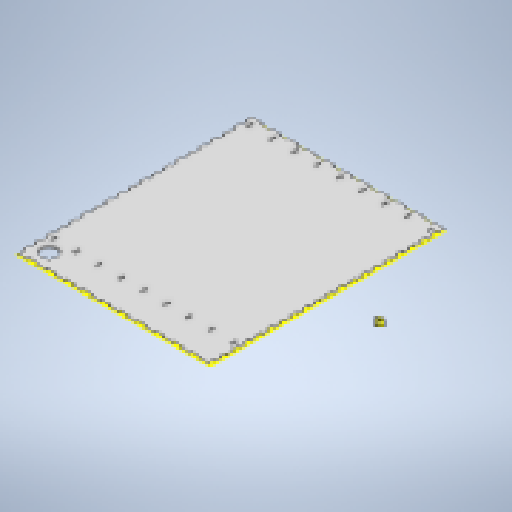
# Autodesk Inventor part: LedBoard
Saved by Autodesk Inventor 2024 (Build 280153000, 153)
## iProperties
Created: 2023-07-20
Part Number: LedBoard
Material: Generic
Document SubType Name: Modeling
Designer: Bruno
Density: 1 g/cm^3
Appearance: Default
Author: Bruno
Autodesk Inventor part; units mm, degrees
ref_plane "YZ Plane" through (0, 0, 0) normal (1, 0, 0) x (0, 1, 0)
ref_plane "XZ Plane" through (0, 0, 0) normal (0, 1, 0) x (-1, 0, 0)
ref_plane "XY Plane" through (0, 0, 0) normal (0, 0, 1) x (1, 0, 0)
sketch "Sketch1" plane through (0, 0, 0) normal (0, 1, 0) x (-1, 0, 0)
  line L0 (378.2704, -187.5) -> (378.2704, 177.5) projected
  line L1 (78.2704, -187.5) -> (378.2704, -187.5) projected
  line L2 (78.2704, 177.5) -> (78.2704, -187.5) projected
  line L3 (378.2704, 177.5) -> (78.2704, 177.5) projected
  line L4 (378.2704, 168.375) -> (378.2704, 177.5) projected
  line L5 (378.2704, 177.5) -> (375.2704, 177.5) projected
  line L6 (375.2704, 168.375) -> (375.2704, 177.5) projected
  line L7 (378.2704, 168.375) -> (375.2704, 168.375) projected
  line L8 (378.2704, 150.125) -> (378.2704, 159.25) projected
  line L9 (378.2704, 159.25) -> (375.2704, 159.25) projected
  line L10 (375.2704, 150.125) -> (375.2704, 159.25) projected
  line L11 (378.2704, 150.125) -> (375.2704, 150.125) projected
  line L12 (378.2704, 131.875) -> (378.2704, 141) projected
  line L13 (378.2704, 141) -> (375.2704, 141) projected
  line L14 (375.2704, 131.875) -> (375.2704, 141) projected
  line L15 (378.2704, 131.875) -> (375.2704, 131.875) projected
  line L16 (378.2704, 113.625) -> (378.2704, 122.75) projected
  line L17 (378.2704, 122.75) -> (375.2704, 122.75) projected
  line L18 (375.2704, 113.625) -> (375.2704, 122.75) projected
  line L19 (378.2704, 113.625) -> (375.2704, 113.625) projected
  line L20 (378.2704, 95.375) -> (378.2704, 104.5) projected
  line L21 (378.2704, 104.5) -> (375.2704, 104.5) projected
  line L22 (375.2704, 95.375) -> (375.2704, 104.5) projected
  line L23 (378.2704, 95.375) -> (375.2704, 95.375) projected
  line L24 (378.2704, 77.125) -> (378.2704, 86.25) projected
  line L25 (378.2704, 86.25) -> (375.2704, 86.25) projected
  line L26 (375.2704, 77.125) -> (375.2704, 86.25) projected
  line L27 (378.2704, 77.125) -> (375.2704, 77.125) projected
  line L28 (378.2704, 58.875) -> (378.2704, 68) projected
  line L29 (378.2704, 68) -> (375.2704, 68) projected
  line L30 (375.2704, 58.875) -> (375.2704, 68) projected
  line L31 (378.2704, 58.875) -> (375.2704, 58.875) projected
  line L32 (378.2704, 4.125) -> (378.2704, 13.25) projected
  line L33 (378.2704, 13.25) -> (375.2704, 13.25) projected
  line L34 (375.2704, 4.125) -> (375.2704, 13.25) projected
  line L35 (378.2704, 4.125) -> (375.2704, 4.125) projected
  line L36 (378.2704, 22.375) -> (378.2704, 31.5) projected
  line L37 (378.2704, 31.5) -> (375.2704, 31.5) projected
  line L38 (375.2704, 22.375) -> (375.2704, 31.5) projected
  line L39 (378.2704, 22.375) -> (375.2704, 22.375) projected
  line L40 (378.2704, 40.625) -> (378.2704, 49.75) projected
  line L41 (378.2704, 49.75) -> (375.2704, 49.75) projected
  line L42 (375.2704, 40.625) -> (375.2704, 49.75) projected
  line L43 (378.2704, 40.625) -> (375.2704, 40.625) projected
  line L44 (378.2704, -87.125) -> (378.2704, -78) projected
  line L45 (378.2704, -78) -> (375.2704, -78) projected
  line L46 (375.2704, -87.125) -> (375.2704, -78) projected
  line L47 (378.2704, -87.125) -> (375.2704, -87.125) projected
  line L48 (378.2704, -68.875) -> (378.2704, -59.75) projected
  line L49 (378.2704, -59.75) -> (375.2704, -59.75) projected
  line L50 (375.2704, -68.875) -> (375.2704, -59.75) projected
  line L51 (378.2704, -68.875) -> (375.2704, -68.875) projected
  line L52 (378.2704, -50.625) -> (378.2704, -41.5) projected
  line L53 (378.2704, -41.5) -> (375.2704, -41.5) projected
  line L54 (375.2704, -50.625) -> (375.2704, -41.5) projected
  line L55 (378.2704, -50.625) -> (375.2704, -50.625) projected
  line L56 (378.2704, -32.375) -> (378.2704, -23.25) projected
  line L57 (378.2704, -23.25) -> (375.2704, -23.25) projected
  line L58 (375.2704, -32.375) -> (375.2704, -23.25) projected
  line L59 (378.2704, -32.375) -> (375.2704, -32.375) projected
  line L60 (378.2704, -14.125) -> (378.2704, -5) projected
  line L61 (378.2704, -5) -> (375.2704, -5) projected
  line L62 (375.2704, -14.125) -> (375.2704, -5) projected
  line L63 (378.2704, -14.125) -> (375.2704, -14.125) projected
  line L64 (378.2704, -178.375) -> (378.2704, -169.25) projected
  line L65 (378.2704, -169.25) -> (375.2704, -169.25) projected
  line L66 (375.2704, -178.375) -> (375.2704, -169.25) projected
  line L67 (378.2704, -178.375) -> (375.2704, -178.375) projected
  line L68 (378.2704, -160.125) -> (378.2704, -151) projected
  line L69 (378.2704, -151) -> (375.2704, -151) projected
  line L70 (375.2704, -160.125) -> (375.2704, -151) projected
  line L71 (378.2704, -160.125) -> (375.2704, -160.125) projected
  line L72 (378.2704, -141.875) -> (378.2704, -132.75) projected
  line L73 (378.2704, -132.75) -> (375.2704, -132.75) projected
  line L74 (375.2704, -141.875) -> (375.2704, -132.75) projected
  line L75 (378.2704, -141.875) -> (375.2704, -141.875) projected
  line L76 (378.2704, -123.625) -> (378.2704, -114.5) projected
  line L77 (378.2704, -114.5) -> (375.2704, -114.5) projected
  line L78 (375.2704, -123.625) -> (375.2704, -114.5) projected
  line L79 (378.2704, -123.625) -> (375.2704, -123.625) projected
  line L80 (378.2704, -105.375) -> (378.2704, -96.25) projected
  line L81 (378.2704, -96.25) -> (375.2704, -96.25) projected
  line L82 (375.2704, -105.375) -> (375.2704, -96.25) projected
  line L83 (378.2704, -105.375) -> (375.2704, -105.375) projected
  line L84 (361.2704, -184.5) -> (347.2704, -184.5) projected
  line L85 (347.2704, -184.5) -> (347.2704, -187.5) projected
  line L86 (361.2704, -187.5) -> (347.2704, -187.5) projected
  line L87 (361.2704, -184.5) -> (361.2704, -187.5) projected
  line L88 (333.2704, -184.5) -> (319.2704, -184.5) projected
  line L89 (319.2704, -184.5) -> (319.2704, -187.5) projected
  line L90 (333.2704, -187.5) -> (319.2704, -187.5) projected
  line L91 (333.2704, -184.5) -> (333.2704, -187.5) projected
  line L92 (305.2704, -184.5) -> (291.2704, -184.5) projected
  line L93 (291.2704, -184.5) -> (291.2704, -187.5) projected
  line L94 (305.2704, -187.5) -> (291.2704, -187.5) projected
  line L95 (305.2704, -184.5) -> (305.2704, -187.5) projected
  line L96 (277.2704, -184.5) -> (263.2704, -184.5) projected
  line L97 (263.2704, -184.5) -> (263.2704, -187.5) projected
  line L98 (277.2704, -187.5) -> (263.2704, -187.5) projected
  line L99 (277.2704, -184.5) -> (277.2704, -187.5) projected
  line L100 (249.2704, -184.5) -> (235.2704, -184.5) projected
  line L101 (235.2704, -184.5) -> (235.2704, -187.5) projected
  line L102 (249.2704, -187.5) -> (235.2704, -187.5) projected
  line L103 (249.2704, -184.5) -> (249.2704, -187.5) projected
  line L104 (221.2704, -184.5) -> (207.2704, -184.5) projected
  line L105 (207.2704, -184.5) -> (207.2704, -187.5) projected
  line L106 (221.2704, -187.5) -> (207.2704, -187.5) projected
  line L107 (221.2704, -184.5) -> (221.2704, -187.5) projected
  line L108 (193.2704, -184.5) -> (179.2704, -184.5) projected
  line L109 (179.2704, -184.5) -> (179.2704, -187.5) projected
  line L110 (193.2704, -187.5) -> (179.2704, -187.5) projected
  line L111 (193.2704, -184.5) -> (193.2704, -187.5) projected
  line L112 (165.2704, -184.5) -> (151.2704, -184.5) projected
  line L113 (151.2704, -184.5) -> (151.2704, -187.5) projected
  line L114 (165.2704, -187.5) -> (151.2704, -187.5) projected
  line L115 (165.2704, -184.5) -> (165.2704, -187.5) projected
  line L116 (137.2704, -184.5) -> (123.2704, -184.5) projected
  line L117 (123.2704, -184.5) -> (123.2704, -187.5) projected
  line L118 (137.2704, -187.5) -> (123.2704, -187.5) projected
  line L119 (137.2704, -184.5) -> (137.2704, -187.5) projected
  line L120 (109.2704, -184.5) -> (95.2704, -184.5) projected
  line L121 (95.2704, -184.5) -> (95.2704, -187.5) projected
  line L122 (109.2704, -187.5) -> (95.2704, -187.5) projected
  line L123 (109.2704, -184.5) -> (109.2704, -187.5) projected
  line L124 (81.2704, -178.375) -> (81.2704, -169.25) projected
  line L125 (81.2704, -169.25) -> (78.2704, -169.25) projected
  line L126 (78.2704, -178.375) -> (78.2704, -169.25) projected
  line L127 (81.2704, -178.375) -> (78.2704, -178.375) projected
  line L128 (81.2704, -160.125) -> (81.2704, -151) projected
  line L129 (81.2704, -151) -> (78.2704, -151) projected
  line L130 (78.2704, -160.125) -> (78.2704, -151) projected
  line L131 (81.2704, -160.125) -> (78.2704, -160.125) projected
  line L132 (81.2704, -141.875) -> (81.2704, -132.75) projected
  line L133 (81.2704, -132.75) -> (78.2704, -132.75) projected
  line L134 (78.2704, -141.875) -> (78.2704, -132.75) projected
  line L135 (81.2704, -141.875) -> (78.2704, -141.875) projected
  line L136 (81.2704, -123.625) -> (81.2704, -114.5) projected
  line L137 (81.2704, -114.5) -> (78.2704, -114.5) projected
  line L138 (78.2704, -123.625) -> (78.2704, -114.5) projected
  line L139 (81.2704, -123.625) -> (78.2704, -123.625) projected
  line L140 (81.2704, -105.375) -> (81.2704, -96.25) projected
  line L141 (81.2704, -96.25) -> (78.2704, -96.25) projected
  line L142 (78.2704, -105.375) -> (78.2704, -96.25) projected
  line L143 (81.2704, -105.375) -> (78.2704, -105.375) projected
  line L144 (81.2704, -87.125) -> (81.2704, -78) projected
  line L145 (81.2704, -78) -> (78.2704, -78) projected
  line L146 (78.2704, -87.125) -> (78.2704, -78) projected
  line L147 (81.2704, -87.125) -> (78.2704, -87.125) projected
  line L148 (81.2704, -68.875) -> (81.2704, -59.75) projected
  line L149 (81.2704, -59.75) -> (78.2704, -59.75) projected
  line L150 (78.2704, -68.875) -> (78.2704, -59.75) projected
  line L151 (81.2704, -68.875) -> (78.2704, -68.875) projected
  line L152 (81.2704, -50.625) -> (81.2704, -41.5) projected
  line L153 (81.2704, -41.5) -> (78.2704, -41.5) projected
  line L154 (78.2704, -50.625) -> (78.2704, -41.5) projected
  line L155 (81.2704, -50.625) -> (78.2704, -50.625) projected
  line L156 (81.2704, -32.375) -> (81.2704, -23.25) projected
  line L157 (81.2704, -23.25) -> (78.2704, -23.25) projected
  line L158 (78.2704, -32.375) -> (78.2704, -23.25) projected
  line L159 (81.2704, -32.375) -> (78.2704, -32.375) projected
  line L160 (81.2704, -14.125) -> (81.2704, -5) projected
  line L161 (81.2704, -5) -> (78.2704, -5) projected
  line L162 (78.2704, -14.125) -> (78.2704, -5) projected
  line L163 (81.2704, -14.125) -> (78.2704, -14.125) projected
  line L164 (81.2704, 4.125) -> (81.2704, 13.25) projected
  line L165 (81.2704, 13.25) -> (78.2704, 13.25) projected
  line L166 (78.2704, 4.125) -> (78.2704, 13.25) projected
  line L167 (81.2704, 4.125) -> (78.2704, 4.125) projected
  line L168 (81.2704, 22.375) -> (81.2704, 31.5) projected
  line L169 (81.2704, 31.5) -> (78.2704, 31.5) projected
  line L170 (78.2704, 22.375) -> (78.2704, 31.5) projected
  line L171 (81.2704, 22.375) -> (78.2704, 22.375) projected
  line L172 (81.2704, 40.625) -> (81.2704, 49.75) projected
  line L173 (81.2704, 49.75) -> (78.2704, 49.75) projected
  line L174 (78.2704, 40.625) -> (78.2704, 49.75) projected
  line L175 (81.2704, 40.625) -> (78.2704, 40.625) projected
  line L176 (81.2704, 58.875) -> (81.2704, 68) projected
  line L177 (81.2704, 68) -> (78.2704, 68) projected
  line L178 (78.2704, 58.875) -> (78.2704, 68) projected
  line L179 (81.2704, 58.875) -> (78.2704, 58.875) projected
  line L180 (81.2704, 77.125) -> (81.2704, 86.25) projected
  line L181 (81.2704, 86.25) -> (78.2704, 86.25) projected
  line L182 (78.2704, 77.125) -> (78.2704, 86.25) projected
  line L183 (81.2704, 77.125) -> (78.2704, 77.125) projected
  line L184 (81.2704, 95.375) -> (81.2704, 104.5) projected
  line L185 (81.2704, 104.5) -> (78.2704, 104.5) projected
  line L186 (78.2704, 95.375) -> (78.2704, 104.5) projected
  line L187 (81.2704, 95.375) -> (78.2704, 95.375) projected
  line L188 (81.2704, 113.625) -> (81.2704, 122.75) projected
  line L189 (81.2704, 122.75) -> (78.2704, 122.75) projected
  line L190 (78.2704, 113.625) -> (78.2704, 122.75) projected
  line L191 (81.2704, 113.625) -> (78.2704, 113.625) projected
  line L192 (81.2704, 131.875) -> (81.2704, 141) projected
  line L193 (81.2704, 141) -> (78.2704, 141) projected
  line L194 (78.2704, 131.875) -> (78.2704, 141) projected
  line L195 (81.2704, 131.875) -> (78.2704, 131.875) projected
  line L196 (81.2704, 150.125) -> (81.2704, 159.25) projected
  line L197 (81.2704, 159.25) -> (78.2704, 159.25) projected
  line L198 (78.2704, 150.125) -> (78.2704, 159.25) projected
  line L199 (81.2704, 150.125) -> (78.2704, 150.125) projected
  line L200 (81.2704, 168.375) -> (81.2704, 177.5) projected
  line L201 (81.2704, 177.5) -> (78.2704, 177.5) projected
  line L202 (78.2704, 168.375) -> (78.2704, 177.5) projected
  line L203 (81.2704, 168.375) -> (78.2704, 168.375) projected
  line L204 (361.2704, 177.5) -> (347.2704, 177.5) projected
  line L205 (347.2704, 177.5) -> (347.2704, 174.5) projected
  line L206 (361.2704, 174.5) -> (347.2704, 174.5) projected
  line L207 (361.2704, 177.5) -> (361.2704, 174.5) projected
  line L208 (333.2704, 177.5) -> (319.2704, 177.5) projected
  line L209 (319.2704, 177.5) -> (319.2704, 174.5) projected
  line L210 (333.2704, 174.5) -> (319.2704, 174.5) projected
  line L211 (333.2704, 177.5) -> (333.2704, 174.5) projected
  line L212 (305.2704, 177.5) -> (291.2704, 177.5) projected
  line L213 (291.2704, 177.5) -> (291.2704, 174.5) projected
  line L214 (305.2704, 174.5) -> (291.2704, 174.5) projected
  line L215 (305.2704, 177.5) -> (305.2704, 174.5) projected
  line L216 (277.2704, 177.5) -> (263.2704, 177.5) projected
  line L217 (263.2704, 177.5) -> (263.2704, 174.5) projected
  line L218 (277.2704, 174.5) -> (263.2704, 174.5) projected
  line L219 (277.2704, 177.5) -> (277.2704, 174.5) projected
  line L220 (249.2704, 177.5) -> (235.2704, 177.5) projected
  line L221 (235.2704, 177.5) -> (235.2704, 174.5) projected
  line L222 (249.2704, 174.5) -> (235.2704, 174.5) projected
  line L223 (249.2704, 177.5) -> (249.2704, 174.5) projected
  line L224 (221.2704, 177.5) -> (207.2704, 177.5) projected
  line L225 (207.2704, 177.5) -> (207.2704, 174.5) projected
  line L226 (221.2704, 174.5) -> (207.2704, 174.5) projected
  line L227 (221.2704, 177.5) -> (221.2704, 174.5) projected
  line L228 (193.2704, 177.5) -> (179.2704, 177.5) projected
  line L229 (179.2704, 177.5) -> (179.2704, 174.5) projected
  line L230 (193.2704, 174.5) -> (179.2704, 174.5) projected
  line L231 (193.2704, 177.5) -> (193.2704, 174.5) projected
  line L232 (165.2704, 177.5) -> (151.2704, 177.5) projected
  line L233 (151.2704, 177.5) -> (151.2704, 174.5) projected
  line L234 (165.2704, 174.5) -> (151.2704, 174.5) projected
  line L235 (165.2704, 177.5) -> (165.2704, 174.5) projected
  line L236 (137.2704, 177.5) -> (123.2704, 177.5) projected
  line L237 (123.2704, 177.5) -> (123.2704, 174.5) projected
  line L238 (137.2704, 174.5) -> (123.2704, 174.5) projected
  line L239 (137.2704, 177.5) -> (137.2704, 174.5) projected
  line L240 (109.2704, 177.5) -> (95.2704, 177.5) projected
  line L241 (95.2704, 177.5) -> (95.2704, 174.5) projected
  line L242 (109.2704, 174.5) -> (95.2704, 174.5) projected
  line L243 (109.2704, 177.5) -> (109.2704, 174.5) projected
  constraints: 4 other
extrude "Extrusion1" add sketch "Sketch1" along normal blind 3 contours L1 L87 L84 L85 L91 L88 L89 L95 L92 L93 L99 L96 L97 L103 L100 L101 L107 L104 L105 L111 L108 L109 L115 L112 L113 L119 L116 L117 L123 L120 L121 L2 L127 L124 L125 L131 L128 L129 L135 L132 L133 L139 L136 L137 L143 L140 L141 L147 L144 L145 L151 L148 L149 L155 L152 L153 L159 L156 L157 L163 L160 L161 L167 L164 L165 L171 L168 L169 L175 L172 L173 L179 L176 L177 L183 L180 L181 L187 L184 L185 L191 L188 L189 L195 L192 L193 L199 L196 L197 L203 L200 L3 L241 L242 L243 L237 L238 L239 L233 L234 L235 L229 L230 L231 L225 L226 L227 L221 L222 L223 L217 L218 L219 L213 L214 L215 L209 L210 L211 L205 L206 L207 L6 L7 L0 L9 L10 L11 L13 L14 L15 L17 L18 L19 L21 L22 L23 L25 L26 L27 L29 L30 L31 L41 L42 L43 L37 L38 L39 L33 L34 L35 L61 L62 L63 L57 L58 L59 L53 L54 L55 L49 L50 L51 L45 L46 L47 L81 L82 L83 L77 L78 L79 L73 L74 L75 L69 L70 L71 L65 L66 L67
sketch "Sketch3" plane through (0, 0, 0) normal (0, -1, 0) x (1, 0, 0)
  line L0 (-369.7704, 134.05) -> (-369.7704, 126.05) projected
  line L1 (-369.7704, 126.05) -> (-366.7704, 126.05) projected
  line L2 (-366.7704, 134.05) -> (-366.7704, 126.05) projected
  line L3 (-369.7704, 134.05) -> (-366.7704, 134.05) projected
  line L4 (-334.7704, 134.05) -> (-334.7704, 126.05) projected
  line L5 (-334.7704, 126.05) -> (-331.7704, 126.05) projected
  line L6 (-331.7704, 134.05) -> (-331.7704, 126.05) projected
  line L7 (-334.7704, 134.05) -> (-331.7704, 134.05) projected
  line L8 (-299.7704, 134.05) -> (-299.7704, 126.05) projected
  line L9 (-299.7704, 126.05) -> (-296.7704, 126.05) projected
  line L10 (-296.7704, 134.05) -> (-296.7704, 126.05) projected
  line L11 (-299.7704, 134.05) -> (-296.7704, 134.05) projected
  line L12 (-264.7704, 134.05) -> (-264.7704, 126.05) projected
  line L13 (-264.7704, 126.05) -> (-261.7704, 126.05) projected
  line L14 (-261.7704, 134.05) -> (-261.7704, 126.05) projected
  line L15 (-264.7704, 134.05) -> (-261.7704, 134.05) projected
  line L16 (-229.7704, 134.05) -> (-229.7704, 126.05) projected
  line L17 (-229.7704, 126.05) -> (-226.7704, 126.05) projected
  line L18 (-226.7704, 134.05) -> (-226.7704, 126.05) projected
  line L19 (-229.7704, 134.05) -> (-226.7704, 134.05) projected
  line L20 (-194.7704, 134.05) -> (-194.7704, 126.05) projected
  line L21 (-194.7704, 126.05) -> (-191.7704, 126.05) projected
  line L22 (-191.7704, 134.05) -> (-191.7704, 126.05) projected
  line L23 (-194.7704, 134.05) -> (-191.7704, 134.05) projected
  line L24 (-159.7704, 134.05) -> (-159.7704, 126.05) projected
  line L25 (-159.7704, 126.05) -> (-156.7704, 126.05) projected
  line L26 (-156.7704, 134.05) -> (-156.7704, 126.05) projected
  line L27 (-159.7704, 134.05) -> (-156.7704, 134.05) projected
  line L28 (-124.7704, 134.05) -> (-124.7704, 126.05) projected
  line L29 (-124.7704, 126.05) -> (-121.7704, 126.05) projected
  line L30 (-121.7704, 134.05) -> (-121.7704, 126.05) projected
  line L31 (-124.7704, 134.05) -> (-121.7704, 134.05) projected
  line L32 (-89.7704, 134.05) -> (-89.7704, 126.05) projected
  line L33 (-89.7704, 126.05) -> (-86.7704, 126.05) projected
  line L34 (-86.7704, 134.05) -> (-86.7704, 126.05) projected
  line L35 (-89.7704, 134.05) -> (-86.7704, 134.05) projected
  line L36 (-369.7704, -171.05) -> (-369.7704, -179.05) projected
  line L37 (-369.7704, -179.05) -> (-366.7704, -179.05) projected
  line L38 (-366.7704, -171.05) -> (-366.7704, -179.05) projected
  line L39 (-369.7704, -171.05) -> (-366.7704, -171.05) projected
  line L40 (-334.7704, -171.05) -> (-334.7704, -179.05) projected
  line L41 (-334.7704, -179.05) -> (-331.7704, -179.05) projected
  line L42 (-331.7704, -171.05) -> (-331.7704, -179.05) projected
  line L43 (-334.7704, -171.05) -> (-331.7704, -171.05) projected
  line L44 (-299.7704, -171.05) -> (-299.7704, -179.05) projected
  line L45 (-299.7704, -179.05) -> (-296.7704, -179.05) projected
  line L46 (-296.7704, -171.05) -> (-296.7704, -179.05) projected
  line L47 (-299.7704, -171.05) -> (-296.7704, -171.05) projected
  line L48 (-264.7704, -171.05) -> (-264.7704, -179.05) projected
  line L49 (-264.7704, -179.05) -> (-261.7704, -179.05) projected
  line L50 (-261.7704, -171.05) -> (-261.7704, -179.05) projected
  line L51 (-264.7704, -171.05) -> (-261.7704, -171.05) projected
  line L52 (-229.7704, -171.05) -> (-229.7704, -179.05) projected
  line L53 (-229.7704, -179.05) -> (-226.7704, -179.05) projected
  line L54 (-226.7704, -171.05) -> (-226.7704, -179.05) projected
  line L55 (-229.7704, -171.05) -> (-226.7704, -171.05) projected
  line L56 (-194.7704, -171.05) -> (-194.7704, -179.05) projected
  line L57 (-194.7704, -179.05) -> (-191.7704, -179.05) projected
  line L58 (-191.7704, -171.05) -> (-191.7704, -179.05) projected
  line L59 (-194.7704, -171.05) -> (-191.7704, -171.05) projected
  line L60 (-159.7704, -171.05) -> (-159.7704, -179.05) projected
  line L61 (-159.7704, -179.05) -> (-156.7704, -179.05) projected
  line L62 (-156.7704, -171.05) -> (-156.7704, -179.05) projected
  line L63 (-159.7704, -171.05) -> (-156.7704, -171.05) projected
  line L64 (-124.7704, -171.05) -> (-124.7704, -179.05) projected
  line L65 (-124.7704, -179.05) -> (-121.7704, -179.05) projected
  line L66 (-121.7704, -171.05) -> (-121.7704, -179.05) projected
  line L67 (-124.7704, -171.05) -> (-121.7704, -171.05) projected
  line L68 (-89.7704, -171.05) -> (-89.7704, -179.05) projected
  line L69 (-89.7704, -179.05) -> (-86.7704, -179.05) projected
  line L70 (-86.7704, -171.05) -> (-86.7704, -179.05) projected
  line L71 (-89.7704, -171.05) -> (-86.7704, -171.05) projected
  point P0 (0, 0)
extrude "Extrusion3" cut sketch "Sketch3" against normal up to surface (3 mm away)
sketch "Sketch4" plane through (0, 3, 0) normal (0, 1, 0) x (1, 0, 0)
  circle A0 centre (-353.2704, -152.5) radius 12.5
  line L0 (-353.2704, -152.5) -> (-378.2704, -152.5) construction
  line L1 (-378.2704, -141) -> (-378.2704, -150.125) projected
  line L2 (-353.2704, -152.5) -> (-353.2704, -177.5) construction
  line L3 (-375.2704, -177.5) -> (-361.2704, -177.5) projected
  point P0 (0, 0)
  point P1 (-78.2704, -177.5)
  dimension "d16" = 25
  dimension "d17" = 25
  dimension "d18" = 25
  constraints: 4 end point, 2 perpendicular, 2 point on line, 1 centre point
  measures "d16" diameter of A0
  measures "d17" distance of L0.start L2.end
  measures "d18" distance of L0.start L0.end
extrude "Extrusion4" cut sketch "Sketch4" against normal through all
body "Solid1"
